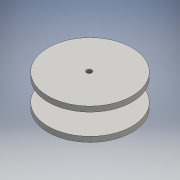
# Autodesk Inventor part: spool model
Saved by Autodesk Inventor 2016 (Build 200138000, 138)
## iProperties
Created: 2015-10-06
Part Number: spool model
Material: Generic
Document SubType Name: Modeling
Designer: phiro
Density: 1 g/cm^3
Appearance: Default
Author: phiro
Autodesk Inventor part; units mm, degrees
ref_plane "YZ Plane" through (0, 0, 0) normal (1, 0, 0) x (0, 1, 0)
ref_plane "XZ Plane" through (0, 0, 0) normal (0, 1, 0) x (-1, 0, 0)
ref_plane "XY Plane" through (0, 0, 0) normal (0, 0, 1) x (1, 0, 0)
sketch "Sketch1" plane through (0, 0, 0) normal (0, 1, 0) x (-1, 0, 0)
  point P0 (0, 0)
sketch "Sketch2" plane through (0, 0, 0) normal (0, 1, 0) x (-1, 0, 0)
  line L0 (-51.7536, 0) -> (-51.7536, -6.35)
  line L1 (-51.7536, -6.35) -> (-0.9536, -6.35)
  line L2 (-0.9536, -6.35) -> (-0.9536, 6.35)
  line L3 (-13.6536, 0) -> (-13.6536, 25.4)
  line L4 (-0.9536, 25.4) -> (-0.9536, 6.35)
  line L5 (-13.6536, 0) -> (-51.7536, 0)
  line L6 (-51.7536, 25.4) -> (-51.7536, 31.75)
  line L7 (-51.7536, 31.75) -> (-0.9536, 31.75)
  line L8 (-0.9536, 31.75) -> (-0.9536, 25.4)
  line L9 (-13.6536, 25.4) -> (-51.7536, 25.4)
  point P0 (0, 0)
  dimension "d0" = 50.8
  dimension "d1" = 6.35
  dimension "d2" = 12.7
  dimension "d3" = 25.4
  dimension "d5" = 6.35
  constraints: 20 end point, 3 parallel, 2 horizontal
  measures "d0" distance of L1.end L0.end
  measures "d1" distance of L0.end L0.start
  measures "d2" distance of L3.end L4.start
  measures "d3" distance of L3.start L3.end
  measures "d5" distance of L6.start L6.end
revolve "Revolution1" add sketch "Sketch2" angle 360 about axis through (0.9536, 0, 25.4) along (0, 0, -1)
sketch "Sketch3" plane through (0.9536, 0, 31.75) normal (0, 0, 1) x (1, 0, 0)
  circle A0 centre (0, 0) radius 50.8 projected
  point P0 (-0.9536, 0)
hole "Hole1" at (0, 0, 31.75) direction (0, 0, -1) diameter 6.35 end through all
body "Solid1"
